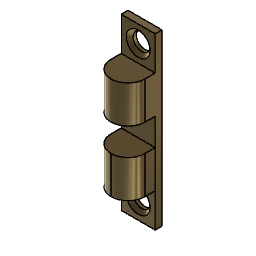
clip_connector_base (Autodesk Fusion 360 design; units mm, degrees)
Autodesk Fusion 360 part; units mm, degrees
sketch "Sketch1" plane through (0, 0, 0) normal (0, 1, 0) x (1, 0, 0)
  line L0 (0, 0) -> (10, 0)
  line L1 (10, 0) -> (10, -50)
  line L2 (10, -50) -> (0, -50)
  line L3 (0, -50) -> (0, 0)
  dimension "d1" = 10
  dimension "d2" = 50
  constraint horizontal L0
  constraint vertical L1
  constraint horizontal L2
  constraint vertical L3
  constraint coincident L0.start L3.end
  measures "d1" distance of L1.end L2.end
  measures "d2" distance of L0.end L1.end
extrude "Extrude1" add sketch "Sketch1" against normal blind 2
sketch "Sketch2" plane through (0, -2, 0) normal (0, -1, 0) x (1, 0, 0)
  line L0 (10, 50) -> (0, 50)
  line L1 (0, 50) -> (0, 0)
  line L2 (0, 0) -> (10, 0)
  line L3 (10, 0) -> (10, 50)
  line L4 (0, 40) -> (10, 40)
  line L5 (10, 40) -> (10, 29)
  line L6 (10, 29) -> (0, 29)
  line L7 (0, 29) -> (0, 40)
  line L8 (0, 10) -> (10, 10)
  line L9 (10, 10) -> (10, 21)
  line L10 (10, 21) -> (0, 21)
  line L11 (0, 21) -> (0, 10)
  circle A0 centre (5, 45) radius 2.5
  circle A1 centre (5, 5) radius 2.5
  dimension "d5" = 5
  dimension "d6" = 5
  dimension "d7" = 5
  dimension "d8" = 5
  dimension "d9" = 11
  dimension "d10" = 11
  dimension "d11" = 10
  dimension "d12" = 10
  dimension "d13" = 8
  dimension "d14" = 5
  dimension "d15" = 5
  dimension "d16" = 5
  constraint horizontal L4
  constraint vertical L5
  constraint horizontal L6
  constraint vertical L7
  constraint coincident L3 L5.end
  constraint coincident L1 L4.start
  constraint horizontal L8
  constraint vertical L9
  constraint horizontal L10
  constraint vertical L11
  constraint coincident L3 L9.end
  constraint coincident L1 L8.start
  measures "d5" distance of L1 A0.centre
  measures "d6" distance of L1 A1.centre
  measures "d7" diameter of A1
  measures "d8" diameter of A0
  measures "d9" distance of L4.end L5.end
  measures "d10" distance of L8.end L9.end
  measures "d11" distance of L0 L4
  measures "d12" distance of L2 L8
  measures "d13" distance of L6 L10
  measures "d14" distance of L4 A0.centre
  measures "d15" distance of L2 A1.centre
  measures "d16" distance of L8 A1.centre
extrude "Extrude2" add sketch "Sketch2" along normal blind 8 contours L1 L3 L4 L5 L6 L7 | L1 L3 L8 L9 L10 L11
extrude "Extrude3" cut sketch "Sketch2" against normal blind 2 contours A0 | A1
chamfer "Chamfer1" distance 1 angle 45 2 edges at (2.6692, -2, 45.904) (2.6692, -2, 5.904)
fillet "Fillet1" radius 5 4 edges at (0, -10, 34.5) (0, -10, 15.5) (10, -10, 34.5) (10, -10, 15.5)
named bodies: "Clip Connector Base"
